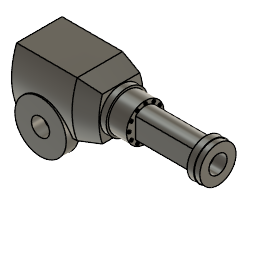
Assembly Of Industrial Robotic Arm (Autodesk Fusion 360 archive; units mm, degrees)
design "Jaw 3"
part number: 2026-06-18-21-04-33-083
Autodesk Fusion 360 part; units mm, degrees
sketch "Sketch1" plane through (0, 0, 0) normal (1, 0, 0) x (0, 1, 0)
  line L0 (0, 0) -> (0, 45)
  line L1 (0, 0) -> (0, -45)
  line L2 (0, 45) -> (37.5, 45)
  line L3 (0, 45) -> (-37.5, 45)
  line L4 (0, -45) -> (37.5, -45)
  line L5 (0, -45) -> (-37.5, -45)
  arc A0 (-37.5, 45) -> (-37.5, -45) centre (79.119, 0) ccw
  arc A1 (37.5, -45) -> (37.5, 45) centre (-79.119, 0) ccw
  dimension "d1" = 37.5
  dimension "d2" = 37.5
  dimension "d3" = 37.5
  dimension "d4" = 37.5
  dimension "d5" = 125
  dimension "d6" = 125
  constraint coincident L0.start L1.start
  constraint vertical L0
  constraint parallel L0 L1
  constraint perpendicular L0 L2
  constraint perpendicular L0 L3
  constraint perpendicular L1 L4
  constraint perpendicular L1 L5
  measures "d1" distance of L0.end L2.end
  measures "d2" distance of L0.end L3.end
  measures "d3" distance of L1.end L4.end
  measures "d4" distance of L1.end L5.end
  measures "d5" radius of A0
  measures "d6" radius of A1
extrude "Extrude1" add sketch "Sketch1" along normal blind 100
extrude "Extrude2" add 1 faces at (100, -15.1807, 3.0661) along direction (1, 0, 0) blind 35 draft -15
sketch "Sketch2" plane through (135, 0, 0) normal (1, 0, 0) x (0, 1, 0)
  line L0 (-30.8786, -35.6218) -> (30.8786, -35.6218)
  arc A0 (30.8786, -35.6218) -> (30.8786, 35.6218) centre (-79.119, 0) ccw
  line L1 (30.8786, 35.6218) -> (-30.8786, 35.6218)
  arc A1 (-30.8786, 35.6218) -> (-30.8786, -35.6218) centre (79.119, 0) ccw
  circle A2 centre (0, 0) radius 34.5
  dimension "d11" = 69
  constraint coincident A2.centre origin
  measures "d11" diameter of A2
extrude "Extrude3" add sketch "Sketch2" along normal blind 10 contours A2
sketch "Sketch3" plane through (145, 0, 0) normal (1, 0, 0) x (0, 1, 0)
  circle A0 centre (0, 0) radius 34.5
  circle A1 centre (0, 0) radius 31
  dimension "d14" = 62
  constraint coincident A0.centre A1.centre
  measures "d14" diameter of A1
extrude "Extrude4" add sketch "Sketch3" along normal blind 30 contours A1
sketch "Sketch4" plane through (175, 0, 0) normal (1, 0, 0) x (0, 1, 0)
  circle A0 centre (0, 0) radius 31
  line L0 (0, 0) -> (27, 0)
  circle A1 centre (27, 0) radius 2.5
  circle A2 centre (27, 0) radius 1.5
  dimension "d17" = 27
  dimension "d18" = 5
  dimension "d19" = -1
  constraint coincident A0.centre L0.start
  constraint horizontal L0
  constraint coincident L0.end A1.centre
  measures "d17" distance of A0.centre L0.end
  measures "d18" diameter of A1
extrude "Extrude5" add sketch "Sketch4" along normal blind 1 contours A1
pattern_circular "C-Pattern1" count 12 over 360 about axis through (175, 0, 0) along (1, 0, 0) of "Extrude5"
sketch "Sketch5" plane through (175, 0, 0) normal (1, 0, 0) x (0, 1, 0)
  circle A0 centre (13.5, -23.3827) radius 2.5
  circle A1 centre (-13.5, -23.3827) radius 2.5
  circle A2 centre (-27, 0) radius 2.5
  circle A3 centre (-13.5, 23.3827) radius 2.5
  circle A4 centre (13.5, 23.3827) radius 2.5
  circle A5 centre (27, 0) radius 2.5
  circle A6 centre (0, 0) radius 31
  circle A7 centre (23.3827, 13.5) radius 2.5
  circle A8 centre (0, 27) radius 2.5
  circle A9 centre (-23.3827, 13.5) radius 2.5
  circle A10 centre (-23.3827, -13.5) radius 2.5
  circle A11 centre (0, -27) radius 2.5
  circle A12 centre (23.3827, -13.5) radius 2.5
  line L0 (16, 0) -> (16, 17)
  line L1 (16, 0) -> (16, -17)
  line L2 (-16, 0) -> (-16, 17)
  line L3 (-16, 0) -> (-16, -17)
  arc A13 (-16, -17) -> (16, -17) centre (0, -1.9003) ccw
  arc A14 (16, 17) -> (-16, 17) centre (0, 1.9003) ccw
  dimension "d32" = 22
  dimension "d33" = 17
  dimension "d34" = 17
  measures "d32" radius of A13
  measures "d33" distance of L0.start L1.end
  measures "d34" distance of L0.start L0.end
extrude "Extrude6" add sketch "Sketch5" along normal blind 100 contours L0 L1 L2 L3 A13 A14
sketch "Sketch6" plane through (275, 0, 0) normal (1, 0, 0) x (0, 1, 0)
  line L0 (16, -17) -> (16, 17)
  arc A0 (16, 17) -> (-16, 17) centre (0, 1.9003) ccw
  line L1 (-16, 17) -> (-16, -17)
  arc A1 (-16, -17) -> (16, -17) centre (0, -1.9003) ccw
  circle A2 centre (0, 0) radius 31
  dimension "d37" = 62
  constraint coincident A2.centre origin
  measures "d37" diameter of A2
extrude "Extrude7" add sketch "Sketch6" along normal blind 10 contours L0 A0 L1 A1 | A2
sketch "Sketch7" plane through (285, 0, 0) normal (1, 0, 0) x (0, 1, 0)
  circle A0 centre (0, 0) radius 31
  circle A1 centre (0, 0) radius 30
  dimension "d40" = -1
extrude "Extrude8" add sketch "Sketch7" along normal blind 1
sketch "Sketch8" plane through (285, 0, 0) normal (1, 0, 0) x (0, 1, 0)
  circle A0 centre (0, 0) radius 30
  circle A1 centre (0, 0) radius 31
  dimension "d43" = 62
  constraint coincident A0.centre A1.centre
  measures "d43" diameter of A1
extrude "Extrude9" add sketch "Sketch8" along normal blind 10 contours A0
ref_plane "WorkPlane1" through (0, -37.5, 45) normal (0, -1, 0) x (1, 0, 0)
sketch "Sketch9" plane through (0, -37.5, 0) normal (0, -1, 0) x (-1, 0, 0)
  circle A0 centre (-50, 45) radius 42.5
  dimension "d46" = 85
  measures "d46" diameter of A0
extrude "Extrude10" add sketch "Sketch9" along normal mid plane 21
sketch "Sketch10" plane through (0, -27, 0) normal (0, 1, 0) x (-1, 0, 0)
  line L0 (-7.5, -45) -> (-92.5, -45)
  arc A0 (-92.5, -45) -> (-7.5, -45) centre (-50, -45) ccw
  line L1 (-50, -45) -> (-50, -75)
  line L2 (-70, -45) -> (-70, -77.2846)
  line L3 (-30, -45) -> (-30, -77.2846)
  arc A1 (-70, -77.2846) -> (-30, -77.2846) centre (-50, -54.924) ccw
  dimension "d49" = 30
  dimension "d50" = 20
  dimension "d51" = -20
  dimension "d52" = 30
  constraint coincident A0.centre L1.start
  constraint perpendicular L0 L1
  measures "d49" distance of A0.centre L1.end
  measures "d52" radius of A1
extrude "Extrude11" add sketch "Sketch10" along normal blind 35 contours L0 L2 L3 A1
sketch "Sketch11" plane through (70, 0, 0) normal (1, 0, 0) x (0, 1, 0)
  line L0 (-27, -45) -> (-27, -77.2846)
  line L1 (-27, -77.2846) -> (8, -77.2846)
  line L2 (8, -77.2846) -> (8, -45)
  line L3 (8, -45) -> (-27, -45)
  line L4 (8, -45) -> (33, -45)
  line L5 (8, -45) -> (8, -87)
  arc A0 (8, -87) -> (33, -45) centre (-21.8393, -40.7981) ccw
  dimension "d55" = 25
  dimension "d56" = 42
  dimension "d57" = 55
  constraint coincident L2.end L3.start
  constraint perpendicular L2 L4
  constraint perpendicular L1 L5
  measures "d55" distance of L2.end L4.end
  measures "d56" distance of L2.end L5.end
  measures "d57" radius of A0
extrude "Extrude12" add sketch "Sketch11" against normal blind 40 contours L2 L4 L5 A0
extrude "Extrude13" cut 1 faces at (33.5817, 8, -83.0165) along direction (0, 1, 0) blind 25
sketch "Sketch12" plane through (295, 0, 0) normal (1, 0, 0) x (0, 1, 0)
  circle A0 centre (0, 0) radius 30
  circle A1 centre (0, 0) radius 15
  dimension "d62" = 30
  constraint coincident A0.centre A1.centre
  measures "d62" diameter of A1
extrude "Extrude14" cut sketch "Sketch12" against normal blind 20 contours A1
sketch "Sketch13" plane through (0, -48, 0) normal (0, -1, 0) x (1, 0, 0)
  circle A0 centre (50, -45) radius 42.5
  circle A1 centre (50, -45) radius 15
  dimension "d65" = 30
  constraint concentric A0 A1
  measures "d65" diameter of A1
extrude "Extrude15" cut sketch "Sketch13" against normal blind 20 contours A1
equation "d47 = ( 21 / 2 ) * 1 mm"

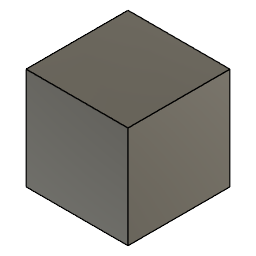
design "Only Object"
part number: 2026-06-24-11-16-10-117
Autodesk Fusion 360 part; units mm, degrees
sketch "Sketch1" plane through (0, 0, 0) normal (0, 0, 1) x (1, 0, 0)
  line L0 (50, -50) -> (-50, -50)
  line L1 (-50, -50) -> (-50, 50)
  line L2 (-50, 50) -> (50, 50)
  line L3 (50, 50) -> (50, -50)
  line L4 (50, -50) -> (-50, 50) construction
  line L5 (-50, -50) -> (50, 50) construction
  dimension "d1" = 100
  dimension "d2" = 100
  constraint horizontal L0
  constraint perpendicular L0 L1
  constraint parallel L0 L2
  constraint parallel L1 L3
  constraint coincident L4 origin
  constraint coincident L5 origin
  measures "d1" distance of L1.end L2.end
  measures "d2" distance of L0.end L1.end
extrude "Extrude1" add sketch "Sketch1" along normal blind 100

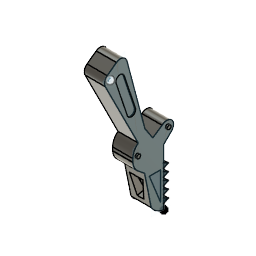
design "Jaw 7"
part number: 2026-06-21-13-52-14-418
Autodesk Fusion 360 part; units mm, degrees
sketch "Sketch1" plane through (0, 0, 0) normal (1, 0, 0) x (0, 1, 0)
  line L0 (486.062, -71.899) -> (454.5004, -9.4181)
  line L1 (454.5004, -9.4181) -> (473.8363, 4.799)
  line L2 (473.8363, 4.799) -> (491.9855, -63.8421)
  line L3 (491.9855, -63.8421) -> (486.062, -71.899)
  line L4 (486.062, -71.899) -> (481.3021, -74.3713)
  line L5 (481.3021, -74.3713) -> (481.3021, -84.3713)
  line L6 (481.3021, -84.3713) -> (481.6163, -89.814)
  line L7 (497.6101, -127.3896) -> (497.6101, -134.3896)
  line L8 (497.6101, -134.3896) -> (508.6101, -134.3896)
  line L9 (508.6101, -134.3896) -> (508.6101, -84.3896)
  line L10 (508.6101, -84.3896) -> (515.6987, -77.3362)
  line L11 (481.6163, -89.814) -> (491.7399, -97.9696)
  line L12 (491.7399, -97.9696) -> (497.6101, -127.3896)
  line L13 (498.9415, -74.4178) -> (507.2345, -68.8298)
  line L14 (491.9855, -63.8421) -> (498.9415, -74.4178)
  arc A0 (515.6987, -77.3362) -> (507.2345, -68.8298) centre (511.4666, -73.083) ccw
  dimension "d1" = 70
  dimension "d2" = 24
  dimension "d3" = 71
  dimension "d4" = 15
  dimension "d5" = 10
  dimension "d6" = 10
  dimension "d7" = 13
  dimension "d8" = 30
  dimension "d9" = 7
  dimension "d10" = 11
  dimension "d11" = 10
  dimension "d12" = 50
  dimension "d14" = 10
  dimension "d15" = 12
  constraint vertical L5
  constraint parallel L5 L7
  constraint perpendicular L7 L8
  constraint perpendicular L8 L9
  constraint tangent L10 A0
  measures "d1" distance of L0.end L0.start
  measures "d2" distance of L0.end L1.end
  measures "d3" distance of L1.end L2.end
  measures "d4" distance of L2.end L4.end
  measures "d5" distance of L2.end L0.start
  measures "d6" distance of L4.end L5.end
  measures "d7" distance of L6.end L11.end
  measures "d8" distance of L7.start L11.end
  measures "d9" distance of L7.start L7.end
  measures "d10" distance of L7.end L8.end
  measures "d11" distance of L9.end L10.end
  measures "d12" distance of L8.end L9.end
  measures "d14" distance of L13.start L13.end
  measures "d15" distance of L10.end L13.end
extrude "Extrude1" add sketch "Sketch1" along normal mid plane 18
sketch "Sketch3" plane through (9, 0, 0) normal (1, 0, 0) x (0, 1, 0)
  line L0 (486.062, -71.899) -> (481.3021, -74.3713)
  line L1 (481.3021, -74.3713) -> (481.3021, -84.3713)
  line L2 (481.3021, -84.3713) -> (481.6163, -89.814)
  line L3 (481.6163, -89.814) -> (491.7399, -97.9696)
  line L4 (491.7399, -97.9696) -> (497.6101, -127.3896)
  line L5 (497.6101, -127.3896) -> (497.6101, -134.3896)
  line L6 (497.6101, -134.3896) -> (508.6101, -134.3896)
  line L7 (508.6101, -134.3896) -> (508.6101, -84.3896)
  line L8 (508.6101, -84.3896) -> (515.6987, -77.3362)
  arc A0 (515.6987, -77.3362) -> (507.2345, -68.8298) centre (511.4666, -73.083) ccw
  line L9 (507.2345, -68.8298) -> (498.9415, -74.4178)
  line L10 (498.9415, -74.4178) -> (491.9855, -63.8421)
  line L11 (491.9855, -63.8421) -> (473.8363, 4.799)
  line L12 (473.8363, 4.799) -> (454.5004, -9.4181)
  line L13 (454.5004, -9.4181) -> (486.062, -71.899)
  line L14 (497.6101, -127.3896) -> (505.9101, -127.3896)
  line L15 (505.9101, -127.3896) -> (505.9101, -102.3896)
  line L16 (505.9101, -102.3896) -> (495.9101, -102.3896)
  line L17 (495.9101, -102.3896) -> (505.9101, -127.3896)
  dimension "d18" = 25
  dimension "d19" = 10
  dimension "d20" = 2.7
  constraint coincident L4.end L5.start
  constraint perpendicular L5 L14
  constraint perpendicular L14 L15
  constraint perpendicular L15 L16
  measures "d18" distance of L14.end L15.end
  measures "d19" distance of L15.end L16.end
  measures "d20" distance of L7 L15
extrude "Extrude2" cut sketch "Sketch3" against normal blind 71 contours L15 L16 L17
sketch "Sketch4" plane through (9, 0, 0) normal (1, 0, 0) x (0, 1, 0)
  line L0 (505.9101, -102.3896) -> (505.9101, -127.3896)
  line L1 (505.9101, -127.3896) -> (495.9101, -102.3896)
  line L2 (495.9101, -102.3896) -> (505.9101, -102.3896)
  line L3 (486.062, -71.899) -> (481.3021, -74.3713)
  line L4 (481.3021, -74.3713) -> (481.3021, -84.3713)
  line L5 (481.3021, -84.3713) -> (481.6163, -89.814)
  line L6 (481.6163, -89.814) -> (491.7399, -97.9696)
  line L7 (491.7399, -97.9696) -> (497.6101, -127.3896)
  line L8 (497.6101, -127.3896) -> (497.6101, -134.3896)
  line L9 (497.6101, -134.3896) -> (508.6101, -134.3896)
  line L10 (508.6101, -134.3896) -> (508.6101, -84.3896)
  line L11 (508.6101, -84.3896) -> (515.6987, -77.3362)
  arc A0 (515.6987, -77.3362) -> (507.2345, -68.8298) centre (511.4666, -73.083) ccw
  line L12 (507.2345, -68.8298) -> (498.9415, -74.4178)
  line L13 (498.9415, -74.4178) -> (491.9855, -63.8421)
  line L14 (491.9855, -63.8421) -> (473.8363, 4.799)
  line L15 (473.8363, 4.799) -> (454.5004, -9.4181)
  line L16 (454.5004, -9.4181) -> (486.062, -71.899)
  line L17 (508.6101, -134.3896) -> (508.6101, -129.3896)
  line L18 (508.6101, -129.3896) -> (508.6101, -125.3896)
  line L19 (508.6101, -127.3896) -> (512.6101, -127.3896)
  line L20 (508.6101, -125.3896) -> (512.6101, -127.3896)
  line L21 (512.6101, -127.3896) -> (508.6101, -129.3896)
  line L22 (508.6101, -118.6396) -> (512.6101, -120.6396)
  line L23 (512.6101, -120.6396) -> (508.6101, -122.6396)
  line L24 (508.6101, -122.6396) -> (508.6101, -118.6396)
  line L25 (508.6101, -111.8896) -> (512.6101, -113.8896)
  line L26 (512.6101, -113.8896) -> (508.6101, -115.8896)
  line L27 (508.6101, -115.8896) -> (508.6101, -111.8896)
  line L28 (508.6101, -105.1396) -> (512.6101, -107.1396)
  line L29 (512.6101, -107.1396) -> (508.6101, -109.1396)
  line L30 (508.6101, -109.1396) -> (508.6101, -105.1396)
  line L31 (508.6101, -98.3896) -> (512.6101, -100.3896)
  line L32 (512.6101, -100.3896) -> (508.6101, -102.3896)
  line L33 (508.6101, -102.3896) -> (508.6101, -98.3896)
  dimension "d23" = 5
  dimension "d24" = 4
  dimension "d25" = 4
  dimension "d30" = 0
  dimension "d31" = 27
  constraint coincident L9.end L10.start
  constraint perpendicular L9 L17
  constraint parallel L10 L18
  constraint midpoint L18 L19.start
  constraint perpendicular L18 L19
  measures "d23" distance of L9.end L17.end
  measures "d24" distance of L17.end L18.end
  measures "d25" distance of L19.start L19.end
extrude "Extrude3" add sketch "Sketch4" against normal up to surface (18 mm away) contours L10 L18 L19 L21 | L10 L18 L19 L20
extrude "Extrude4" add sketch "Sketch4" against normal up to surface (18 mm away) contours L10 L31 L32 L33 | L10 L28 L29 L30 | L10 L22 L23 L24 | L10 L25 L26 L27
fillet "Fillet1" radius 6 2 edges at (0, 473.8363, 4.799) (0, 454.5004, -9.4181)
fillet "Fillet2" radius 15 1 edges at (0, 497.6101, -134.3896)
fillet "Fillet3" radius 12 2 edges at (0, 481.3021, -74.3713) (0, 481.6163, -89.814)
sketch "Sketch5" plane through (9, 0, 0) normal (1, 0, 0) x (0, 1, 0)
  arc A0 (481.3095, -84.5001) -> (485.7614, -93.1532) centre (493.2896, -83.8084) ccw
  line L0 (485.7614, -93.1532) -> (491.7399, -97.9696)
  line L1 (491.7399, -97.9696) -> (497.6101, -127.3896)
  arc A1 (497.6101, -127.3896) -> (508.6101, -134.3896) centre (510.3629, -119.4924) ccw
  line L2 (508.6101, -134.3896) -> (508.6101, -129.3896)
  line L3 (508.6101, -129.3896) -> (512.6101, -127.3896)
  line L4 (512.6101, -127.3896) -> (508.6101, -125.3896)
  line L5 (508.6101, -125.3896) -> (508.6101, -122.6396)
  line L6 (508.6101, -122.6396) -> (512.6101, -120.6396)
  line L7 (512.6101, -120.6396) -> (508.6101, -118.6396)
  line L8 (508.6101, -118.6396) -> (508.6101, -115.8896)
  line L9 (508.6101, -115.8896) -> (512.6101, -113.8896)
  line L10 (512.6101, -113.8896) -> (508.6101, -111.8896)
  line L11 (508.6101, -111.8896) -> (508.6101, -109.1396)
  line L12 (508.6101, -109.1396) -> (512.6101, -107.1396)
  line L13 (512.6101, -107.1396) -> (508.6101, -105.1396)
  line L14 (508.6101, -105.1396) -> (508.6101, -102.3896)
  line L15 (508.6101, -102.3896) -> (512.6101, -100.3896)
  line L16 (512.6101, -100.3896) -> (508.6101, -98.3896)
  line L17 (508.6101, -98.3896) -> (508.6101, -84.3896)
  line L18 (508.6101, -84.3896) -> (515.6987, -77.3362)
  arc A2 (515.6987, -77.3362) -> (507.2345, -68.8298) centre (511.4666, -73.083) ccw
  line L19 (507.2345, -68.8298) -> (498.9415, -74.4178)
  line L20 (498.9415, -74.4178) -> (491.9855, -63.8421)
  line L21 (491.9855, -63.8421) -> (476.0895, -3.7229)
  arc A3 (476.0895, -3.7229) -> (466.7346, -0.4226) centre (470.2889, -5.2566) ccw
  line L22 (466.7346, -0.4226) -> (458.5908, -6.4105)
  arc A4 (458.5908, -6.4105) -> (456.7896, -13.9498) centre (462.1451, -11.2445) ccw
  line L23 (456.7896, -13.9498) -> (486.062, -71.899)
  arc A5 (486.062, -71.899) -> (481.3021, -81.4688) centre (493.3021, -81.4688) ccw
  line L24 (481.3021, -81.4688) -> (481.3021, -84.3713)
  line L25 (481.3021, -84.3713) -> (481.3095, -84.5001)
  line L26 (505.9101, -102.3896) -> (505.9101, -127.3896)
  line L27 (505.9101, -127.3896) -> (495.9101, -102.3896)
  line L28 (495.9101, -102.3896) -> (505.9101, -102.3896)
  circle A6 centre (461, -11) radius 1.5
  dimension "d40" = 3
  measures "d40" diameter of A6
extrude "Extrude5" cut sketch "Sketch5" against normal blind 33 contours A6
sketch "Sketch7" plane through (0, 454.1129, 90.609) normal (0, -0.980669, -0.195673) x (1, 0, 0)
  line L0 (-9, -222.2957) -> (9, -222.2957)
  line L1 (9, -222.2957) -> (9, -192.2957)
  line L2 (9, -192.2957) -> (-9, -192.2957)
  line L3 (-9, -192.2957) -> (-9, -222.2957)
  line L4 (-6, -199.7367) -> (6, -199.7367)
  line L5 (6, -199.7367) -> (9, -199.7367)
  line L6 (-6, -199.7367) -> (-9, -199.7367)
  line L7 (3.1939, -218.0429) -> (-2.6041, -218.0429)
  line L8 (-6, -199.7367) -> (-2.6041, -218.0429)
  line L9 (6, -199.7367) -> (3.1939, -218.0429)
  dimension "d43" = 3
  dimension "d44" = 3
  dimension "d45" = 7.441
  constraint parallel L0 L4
  constraint coincident L1 L5.end
  constraint perpendicular L1 L5
  constraint coincident L3 L6.end
  constraint perpendicular L3 L6
  constraint parallel L4 L7
  measures "d43" distance of L4.start L6.end
  measures "d44" distance of L4.end L5.end
  measures "d45" distance of L2 L4
extrude "Extrude6" cut sketch "Sketch7" against normal blind 9 contours L4 L7 L8 L9
sketch "Sketch8" plane through (9, 0, 0) normal (1, 0, 0) x (0, 1, 0)
  circle A0 centre (512, -72) radius 1.75
  circle A1 centre (485, -81) radius 1.75
  dimension "d48" = 3.5
  dimension "d49" = 3.5
  measures "d48" diameter of A0
  measures "d49" diameter of A1
extrude "Extrude7" add sketch "Sketch8" along normal blind 1.5
sketch "Sketch9" plane through (9, 0, 0) normal (1, 0, 0) x (0, 1, 0)
  line L0 (466.432, -16.1893) -> (476.432, -46.1893)
  arc A0 (476.432, -46.1893) -> (483.568, -43.8107) centre (480, -45) ccw
  line L1 (483.568, -43.8107) -> (473.568, -13.8107)
  arc A1 (473.568, -13.8107) -> (466.432, -16.1893) centre (470, -15) ccw
  line L2 (470, -15) -> (480, -45) construction
  dimension "d52" = 7.522
  constraint tangent L0 A0
  constraint tangent A0 L1
  constraint parallel L0 L1
  constraint tangent L1 A1
  constraint tangent L0 A1
  measures "d52" diameter of A0
extrude "Extrude8" cut sketch "Sketch9" against normal blind 1
ref_plane "WorkPlane1" through (0, 487.2262, -64.7953) normal (-1, 0, 0) x (0, -1, 0)
mirror "Mirror1" about plane through (0, 487.2262, -64.7953) normal (-1, 0, 0) of "Extrude7", "Extrude8"

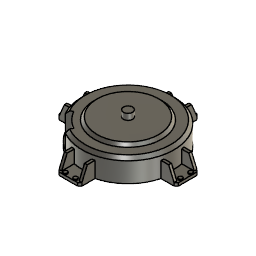
design "Untitled"
part number: 2026-06-13-06-54-28-118
Autodesk Fusion 360 part; units mm, degrees
sketch "Sketch1" plane through (0, 0, 0) normal (0, 0, 1) x (1, 0, 0)
  circle A0 centre (0, 0) radius 150
  dimension "d1" = 300
  constraint coincident A0.centre origin
  measures "d1" diameter of A0
extrude "Extrude1" add sketch "Sketch1" along normal blind 75
chamfer "Chamfer1" distance 10 angle 45 1 edges at (-139.8491, -54.2423, 75)
sketch "Sketch2" plane through (0, 0, 0) normal (0, 0, -1) x (1, 0, 0)
  circle A0 centre (0, 0) radius 150
  circle A1 centre (0, 0) radius 150
  line L0 (-195.2369, -37.5) -> (-145.2369, -37.5)
  line L1 (-110, -50) -> (-110, 50)
  line L2 (-145.2369, 37.5) -> (-195.2369, 37.5)
  line L3 (-195.2369, 37.5) -> (-195.2369, -37.5)
  line L4 (0, 0) -> (-150, 0)
  dimension "d5" = 75
  dimension "d6" = 50
  constraint concentric A0 A1
  constraint horizontal L0
  constraint vertical L1
  constraint horizontal L2
  constraint vertical L3
  constraint coincident A0.centre A1.centre
  constraint coincident A1 L4.end
  constraint perpendicular L1 L4
  constraint symmetric L0 L2 L4
  constraint coincident A0 L0.end
  constraint coincident A0 L2.start
  measures "d5" distance of L0.start L2.end
  measures "d6" distance of L0.start L0.end
extrude "Extrude2" add sketch "Sketch2" against normal blind 10 contours A0 A1 L0 L2 L3
chamfer "Chamfer2" distance 7 angle 45 2 edges at (-195.2369, -37.5, 5) (-195.2369, 37.5, 5)
sketch "Sketch3" plane through (0, -37.5, 0) normal (0, -1, 0) x (1, 0, 0)
  line L0 (-188.2369, 10) -> (-188.2369, 0)
  line L1 (-188.2369, 0) -> (-145.2369, 0)
  line L2 (-145.2369, 0) -> (-145.2369, 10)
  line L3 (-145.2369, 10) -> (-188.2369, 10)
  line L4 (-145.2369, 10) -> (-145.2369, 51.8473)
  line L5 (-145.2369, 51.8473) -> (-170.5569, 51.8473)
  line L6 (-170.5569, 51.8473) -> (-188.2369, 10)
  dimension "d10" = 17.68
  constraint coincident L2.end L3.start
  constraint perpendicular L3 L4
  constraint perpendicular L4 L5
  constraint coincident L0.start L3.end
  measures "d10" horizontal distance of L5.end L0.start
extrude "Extrude3" add sketch "Sketch3" against normal blind 9 contours L3 L4 L5 L6
sketch "Sketch4" plane through (0, 0, 10) normal (0, 0, 1) x (-1, 0, 0)
  line L0 (188.2369, 28.5) -> (147.2676, 28.5)
  arc A0 (145.2369, -37.5) -> (147.2676, 28.5) centre (0, 0) ccw
  line L1 (145.2369, -37.5) -> (188.2369, -37.5)
  line L2 (188.2369, -37.5) -> (195.2369, -30.5)
  line L3 (195.2369, -30.5) -> (195.2369, 30.5)
  line L4 (195.2369, 30.5) -> (188.2369, 37.5)
  line L5 (188.2369, 37.5) -> (188.2369, 28.5)
  line L6 (188.2369, 28.5) -> (188.2369, -37.5)
  line L7 (188.3004, 9.6842) -> (194.2684, 13.2032)
  line L8 (194.2684, 13.2032) -> (194.2049, 20.1311)
  line L9 (194.2049, 20.1311) -> (188.1733, 23.54)
  line L10 (188.1733, 23.54) -> (182.2054, 20.021)
  line L11 (182.2054, 20.021) -> (182.2689, 13.0931)
  line L12 (182.2689, 13.0931) -> (188.3004, 9.6842)
  point P0 (188.2369, 16.6121)
  dimension "d13" = 6
  dimension "d14" = 4.96
  constraint coincident L0.start L5.end
  constraint coincident L1.end L2.start
  constraint coincident L6 P0
  measures "d13" distance of P0 L12
  measures "d14" vertical distance of L0.start L9.end
extrude "Extrude4" add sketch "Sketch4" along normal blind 3.5 contours L6 L7 L8 L9 L12 | L6 L9 L10 L11 L12
ref_plane "WorkPlane1" through (-166.7369, 0, 25.9236) normal (0, -1, 0) x (1, 0, 0)
mirror "Mirror1" about plane through (-166.7369, 0, 25.9236) normal (0, -1, 0) of "Extrude3", "Extrude4"
pattern_circular "C-Pattern1" count 4 over 360 about axis through (0, 0, 1.75) along (0, 0, 1) of "Extrude2", "Chamfer2", "Extrude3", "Extrude4", "Mirror1"
sketch "Sketch5" plane through (0, 0, 75) normal (0, 0, 1) x (-1, 0, 0)
  circle A0 centre (0, 0) radius 140
  line L0 (0, 0) -> (0, 150)
  line L1 (0, 0) -> (150, 0)
  line L2 (0, 0) -> (193.4752, 111.703)
  line L3 (0, 0) -> (90.7609, 157.2025)
  circle A1 centre (0, 0) radius 130
  circle A2 centre (0, 0) radius 150
  dimension "d21" = 30
  dimension "d22" = 30
  dimension "d23" = 260
  dimension "d24" = 300
  constraint coincident A0.centre L0.start
  constraint vertical L0
  constraint perpendicular L0 L1
  measures "d21" angle of L1 L2
  measures "d22" angle of L0 L3
  measures "d23" diameter of A1
  measures "d24" diameter of A2
extrude "Extrude5" cut sketch "Sketch5" against normal blind 60 contours A0 L2 L3 A1 | A0 L2 L3 A2
sketch "Sketch6" plane through (0, 0, 75) normal (0, 0, 1) x (-1, 0, 0)
  line L0 (65, 112.5833) -> (70, 121.2436)
  arc A0 (70, 121.2436) -> (121.2436, 70) centre (0, 0) ccw
  line L1 (121.2436, 70) -> (112.5833, 65)
  arc A1 (112.5833, 65) -> (65, 112.5833) centre (0, 0) ccw
  circle A2 centre (0, 0) radius 110
  dimension "d27" = 220
  constraint concentric A0 A2
  measures "d27" diameter of A2
extrude "Extrude6" add sketch "Sketch6" along normal blind 9 draft -45 contours A2
sketch "Sketch7" plane through (0, 0, 84) normal (0, 0, 1) x (-1, 0, 0)
  circle A0 centre (0, 0) radius 101
  circle A1 centre (0, 0) radius 15
  dimension "d30" = 30
  constraint coincident A0.centre A1.centre
  measures "d30" diameter of A1
extrude "Extrude7" add sketch "Sketch7" along normal blind 20 contours A1

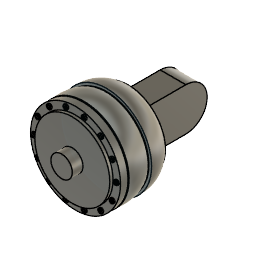
design "Jaw 5"
part number: 2026-06-19-10-47-47-471
Autodesk Fusion 360 part; units mm, degrees
sketch "Sketch1" plane through (0, 0, 0) normal (0, 0, 1) x (1, 0, 0)
  line L0 (0, 0) -> (-35, 0)
  line L1 (0, 0) -> (0, -20)
  line L2 (0, -20) -> (-42, -20)
  arc A0 (-35, 0) -> (-42, -20) centre (-17.1273, -17.4804) ccw
  dimension "d1" = 35
  dimension "d2" = 20
  dimension "d3" = 42
  dimension "d4" = 25
  constraint coincident L0.start L1.start
  constraint horizontal L0
  constraint perpendicular L0 L1
  constraint perpendicular L1 L2
  measures "d1" distance of L0.start L0.end
  measures "d2" distance of L0.start L1.end
  measures "d3" distance of L1.end L2.end
  measures "d4" radius of A0
revolve "Revolve1" add sketch "Sketch1" angle 360 about axis through (0, 0, 0) along (0, -1, 0)
sketch "Sketch2" plane through (0, -20, 0) normal (0, -1, 0) x (1, 0, 0)
  circle A0 centre (0, 0) radius 42
sketch "Sketch3" plane through (0, -20, 0) normal (0, -1, 0) x (1, 0, 0)
  circle A0 centre (0, 0) radius 39.5
  dimension "d6" = 79
  constraint coincident A0.centre origin
  measures "d6" diameter of A0
extrude "Extrude1" add sketch "Sketch3" along normal blind 1
sketch "Sketch4" plane through (0, 0, 0) normal (0, 0, 1) x (1, 0, 0)
  line L0 (0, -21) -> (0, -41)
  line L1 (0, -41) -> (-42, -41)
  line L2 (0, -21) -> (-40, -21)
  arc A0 (-40, -21) -> (-42, -41) centre (-5.5677, -34.5432) ccw
  dimension "d9" = 20
  dimension "d10" = 42
  dimension "d11" = 40
  dimension "d12" = 37
  constraint vertical L0
  constraint perpendicular L0 L1
  constraint perpendicular L0 L2
  measures "d9" distance of L0.start L0.end
  measures "d10" distance of L0.end L1.end
  measures "d11" distance of L0.start L2.end
  measures "d12" radius of A0
revolve "Revolve2" add sketch "Sketch4" angle 360 about axis through (0, -21, 0) along (0, -1, 0)
sketch "Sketch5" plane through (0, -41, 0) normal (0, -1, 0) x (1, 0, 0)
  circle A0 centre (0, 0) radius 42
  circle A1 centre (0, 0) radius 41.25
  dimension "d14" = 82.5
  constraint concentric A0 A1
  measures "d14" diameter of A1
extrude "Extrude2" add sketch "Sketch5" along normal blind 1 contours A1
sketch "Sketch6" plane through (0, -42, 0) normal (0, -1, 0) x (1, 0, 0)
  circle A0 centre (0, 0) radius 41.25
  circle A1 centre (0, 0) radius 42
  dimension "d17" = 84
  constraint coincident A0.centre A1.centre
  measures "d17" diameter of A1
extrude "Extrude3" add sketch "Sketch6" along normal blind 7 contours A0 | A1
sketch "Sketch7" plane through (0, -49, 0) normal (0, -1, 0) x (1, 0, 0)
  circle A0 centre (0, 0) radius 42
  circle A1 centre (0, 0) radius 35
  dimension "d20" = 70
  constraint concentric A0 A1
  measures "d20" diameter of A1
extrude "Extrude4" add sketch "Sketch7" along normal blind 3 contours A1
sketch "Sketch8" plane through (0, -49, 0) normal (0, -1, 0) x (1, 0, 0)
  circle A0 centre (0, 0) radius 35
  circle A1 centre (0, 0) radius 42
  line L0 (35, 0) -> (42, 0)
  circle A2 centre (38.5, 0) radius 2.25
  circle A3 centre (38.5, 0) radius 1.5
  dimension "d23" = 4.5
  dimension "d24" = 3
  constraint coincident A0 L0.start
  constraint coincident A1 L0.end
  constraint horizontal L0
  constraint midpoint L0 A2.centre
  constraint concentric A2 A3
  measures "d23" diameter of A2
  measures "d24" diameter of A3
extrude "Extrude5" add sketch "Sketch8" along normal blind 1 contours L0 A2 A3 | L0 A2 A3
pattern_circular "C-Pattern1" count 14 over 360 about axis through (0, -52, 0) along (0, -1, 0) of "Extrude5"
sketch "Sketch9" plane through (0, 0, 0) normal (0, 1, 0) x (1, 0, 0)
  line L0 (-12, 20) -> (12, 20)
  line L1 (12, 20) -> (12, -20)
  line L2 (12, -20) -> (-12, -20)
  line L3 (-12, -20) -> (-12, 20)
  line L4 (-12, 20) -> (12, -20) construction
  line L5 (12, 20) -> (-12, -20) construction
  dimension "d29" = 24
  dimension "d30" = 40
  constraint horizontal L0
  constraint perpendicular L0 L1
  constraint parallel L0 L2
  constraint parallel L1 L3
  constraint coincident L4 origin
  constraint coincident L5 origin
  measures "d29" distance of L1.end L2.end
  measures "d30" distance of L0.end L1.end
extrude "Extrude6" add sketch "Sketch9" along normal blind 42
sketch "Sketch10" plane through (-12, 0, 0) normal (-1, 0, 0) x (0, -1, 0)
  line L0 (0, -20) -> (0, 20)
  line L1 (0, 20) -> (-42, 20)
  line L2 (-42, 20) -> (-42, -20)
  line L3 (-42, -20) -> (0, -20)
  circle A0 centre (-42, 0) radius 20
  dimension "d33" = 40
  constraint midpoint L2 A0.centre
  measures "d33" diameter of A0
extrude "Extrude7" add sketch "Sketch10" against normal blind 24 contours L2 A0 picked at (-48.2058, -2.4356)
sketch "Sketch11" plane through (-12, 0, 0) normal (-1, 0, 0) x (0, -1, 0)
  line L0 (0, -20) -> (0, 20)
  line L1 (0, 20) -> (-42, 20)
  arc A0 (-42, 20) -> (-42, -20) centre (-42, 0) ccw
  line L2 (-42, -20) -> (0, -20)
  circle A1 centre (-42, 0) radius 10
  dimension "d36" = 20
  constraint concentric A0 A1
  measures "d36" diameter of A1
extrude "Extrude8" add sketch "Sketch11" along normal blind 10 contours A1
sketch "Sketch12" plane through (0, -52, 0) normal (0, -1, 0) x (1, 0, 0)
  circle A0 centre (0, 0) radius 35
  circle A1 centre (0, 0) radius 10
  dimension "d39" = 20
  constraint concentric A0 A1
  measures "d39" diameter of A1
extrude "Extrude9" add sketch "Sketch12" along normal blind 10 contours A1

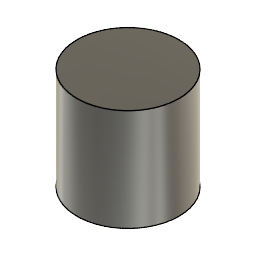
design "Pillar Object"
part number: 2026-06-23-20-36-53-735
Autodesk Fusion 360 part; units mm, degrees
sketch "Sketch1" plane through (0, 0, 0) normal (0, 0, 1) x (1, 0, 0)
  circle A0 centre (0, 0) radius 100
  dimension "d9" = 200
  constraint coincident A0.centre origin
  measures "d9" diameter of A0
extrude "Extrude1" add sketch "Sketch1" along normal blind 200

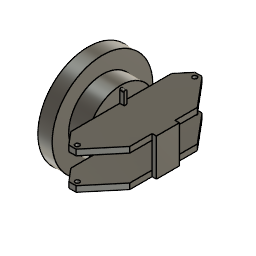
design "Jaw 6"
part number: 2026-06-21-13-07-49-301
Autodesk Fusion 360 part; units mm, degrees
sketch "Sketch1" plane through (0, 0, 0) normal (1, 0, 0) x (0, 1, 0)
  circle A0 centre (0, 0) radius 35
  dimension "d1" = 70
  constraint coincident A0.centre origin
  measures "d1" diameter of A0
extrude "Extrude1" add sketch "Sketch1" along normal blind 10
sketch "Sketch2" plane through (10, 0, 0) normal (1, 0, 0) x (0, 1, 0)
  circle A0 centre (0, 0) radius 35
  circle A1 centre (0, 0) radius 23.5
  dimension "d4" = 47
  constraint coincident A0.centre A1.centre
  measures "d4" diameter of A1
extrude "Extrude2" add sketch "Sketch2" along normal blind 13 contours A1
ref_plane "WorkPlane1" through (0, 0, 13) normal (0, 0, 1) x (1, 0, 0)
sketch "Sketch3" plane through (0, 0, 13) normal (0, 0, 1) x (1, 0, 0)
  line L0 (23, 0) -> (23, -35)
  line L1 (23, -35) -> (23, -45)
  line L2 (23, -35) -> (30.3921, -43.8095)
  line L3 (30.3921, -43.8095) -> (35.3921, -43.8095)
  line L4 (23, 0) -> (60, 0)
  line L5 (23, -23.5) -> (67, -23.5)
  line L6 (35.3921, -43.8095) -> (52.4338, -23.5)
  line L7 (35.3921, -43.8095) -> (47, -43.8095)
  line L8 (52.4338, -23.5) -> (52.4338, 0)
  line L9 (23, 0) -> (23, 35)
  line L10 (23, 35) -> (30.3921, 43.8095)
  line L11 (30.3921, 43.8095) -> (35.3921, 43.8095)
  line L12 (35.3921, 43.8095) -> (52.4338, 23.5)
  line L13 (52.4338, 23.5) -> (52.4338, 0)
  dimension "d8" = 35
  dimension "d9" = 10
  dimension "d10" = 11.5
  dimension "d11" = 40
  dimension "d12" = 5
  dimension "d13" = 50
  constraint vertical L0
  constraint parallel L0 L1
  constraint horizontal L3
  constraint perpendicular L0 L4
  constraint coincident L0 L5.start
  constraint perpendicular L0 L5
  constraint coincident L5 L6.end
  constraint parallel L3 L7
  constraint coincident L4 L8.end
  constraint perpendicular L4 L8
  constraint symmetric L0.start L4 L9.start
  constraint symmetric L0.end L4 L9.end
  constraint symmetric L2.end L4 L10.end
  constraint symmetric L3.end L4 L11.end
  constraint symmetric L4 L6.end L12.end
  constraint symmetric L4 L8.end L13.end
  measures "d8" distance of L0.start L0.end
  measures "d9" distance of L0.end L1.end
  measures "d10" distance of L0.end L2.end
  measures "d11" angle of L1 L2
  measures "d12" distance of L2.end L3.end
  measures "d13" angle of L6 L7
extrude "Extrude3" add sketch "Sketch3" against normal blind 4
sketch "Sketch4" plane through (0, 0, 13) normal (0, 0, 1) x (-1, 0, 0)
  line L0 (-23, -35) -> (-23, -19.5768)
  line L1 (-23, -19.5768) -> (-23, 19.5768)
  line L2 (-23, 19.5768) -> (-23, 35)
  line L3 (-23, 35) -> (-30.3921, 43.8095)
  line L4 (-30.3921, 43.8095) -> (-35.3921, 43.8095)
  line L5 (-35.3921, 43.8095) -> (-52.4338, 23.5)
  line L6 (-52.4338, 23.5) -> (-52.4338, -23.5)
  line L7 (-52.4338, -23.5) -> (-35.3921, -43.8095)
  line L8 (-35.3921, -43.8095) -> (-30.3921, -43.8095)
  line L9 (-30.3921, -43.8095) -> (-23, -35)
  line L10 (-33.3297, 43.8095) -> (-33.3297, 40.8095)
  circle A0 centre (-33.3297, 40.8095) radius 1.5
  dimension "d16" = 3
  dimension "d17" = 3
  constraint coincident L4 L10.start
  constraint perpendicular L4 L10
  constraint coincident L10.end A0.centre
  measures "d16" distance of L10.start L10.end
  measures "d17" diameter of A0
extrude "Extrude4" cut sketch "Sketch4" against normal blind 8 contours A0
mirror "Mirror1" about plane through (0, 0, 0) normal (0, 1, 0) of "Extrude4"
mirror "Mirror2" about plane through (0, 0, 0) normal (0, 0, 1) of "Extrude3", "Extrude4", "Mirror1"
sketch "Sketch5" plane through (23, 0, 0) normal (1, 0, 0) x (0, 1, 0)
  line L0 (-19.5768, 13) -> (19.5768, 13)
  arc A0 (19.5768, 13) -> (-19.5768, 13) centre (0, 0) ccw
  line L1 (0, 13) -> (0, 23.5)
  line L2 (0, 13) -> (-1, 13)
  line L3 (-1, 13) -> (-1, 22)
  line L4 (-1, 22) -> (1, 22)
  line L5 (1, 22) -> (1, 13)
  dimension "d24" = 1
  dimension "d25" = 9
  dimension "d26" = 2
  dimension "d27" = 9
  constraint midpoint L0 L1.start
  constraint midpoint A0 L1.end
  constraint perpendicular L1 L2
  constraint perpendicular L2 L3
  constraint perpendicular L1 L4
  constraint perpendicular L4 L5
  measures "d24" distance of L1.start L2.end
  measures "d25" distance of L2.end L3.end
  measures "d26" distance of L3.end L4.end
  measures "d27" distance of L4.end L5.end
extrude "Extrude5" add sketch "Sketch5" along normal blind 3 contours L0 L1 L2 L3 L4 | L0 L1 L4 L5
fillet "Fillet1" radius 1 2 edges at (24.5, 1, 22) (24.5, -1, 22)
mirror "Mirror3" about plane through (0, 0, 0) normal (0, 0, 1) of "Extrude5", "Fillet1"
sketch "Sketch6" plane through (52.4338, 0, 0) normal (1, 0, 0) x (0, 1, 0)
  line L0 (23.5, 13) -> (-23.5, 13)
  line L1 (-23.5, 13) -> (-23.5, 9)
  line L2 (-23.5, 9) -> (23.5, 9)
  line L3 (23.5, 9) -> (23.5, 13)
  line L4 (8, -13) -> (-8, -13)
  line L5 (-8, -13) -> (-8, 13)
  line L6 (-8, 13) -> (8, 13)
  line L7 (8, 13) -> (8, -13)
  line L8 (8, -13) -> (-8, 13) construction
  line L9 (-8, -13) -> (8, 13) construction
  constraint horizontal L4
  constraint perpendicular L4 L5
  constraint parallel L4 L6
  constraint parallel L5 L7
  constraint coincident L8 origin
  constraint coincident L9 origin
extrude "Extrude6" add sketch "Sketch6" along normal blind 3 contours L0 L2 L5 L6 L7 | L2 L4 L5 L7
sketch "Sketch7" plane through (0, 0, 0) normal (-1, 0, 0) x (0, -1, 0)
  circle A0 centre (0, 0) radius 35
  circle A1 centre (0, 0) radius 10
  dimension "d36" = 20
  constraint coincident A0.centre A1.centre
  measures "d36" diameter of A1
extrude "Extrude7" cut sketch "Sketch7" against normal blind 10 contours A1
